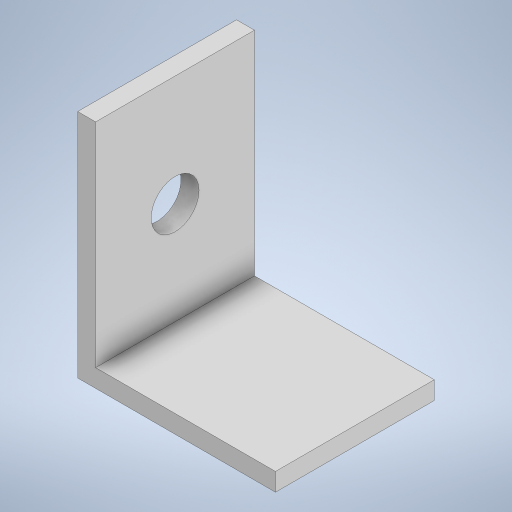
# Autodesk Inventor part: MotorHalterNeu
Saved by Autodesk Inventor 2023 (Build 270158000, 158)
## iProperties
Created: 2024-02-23
Part Number: MotorHalterNeu
Material: Generisch
Document SubType Name: Modeling
Designer: phili
Density: 1 g/cm^3
Appearance: Vorgabe
Author: phili
Autodesk Inventor part; units mm, degrees
ref_plane "YZ Plane" through (0, 0, 0) normal (1, 0, 0) x (0, 1, 0)
ref_plane "XZ Plane" through (0, 0, 0) normal (0, 1, 0) x (-1, 0, 0)
ref_plane "XY Plane" through (0, 0, 0) normal (0, 0, 1) x (1, 0, 0)
sketch "Skizze1" plane through (0, 0, 0) normal (1, 0, 0) x (0, 1, 0)
  line L0 (-19.25, -13.25) -> (19.25, -13.25)
  line L1 (19.25, -13.25) -> (19.25, 13.25)
  line L2 (19.25, 13.25) -> (-19.25, 13.25)
  line L3 (-19.25, 13.25) -> (-19.25, -13.25)
  line L4 (-19.25, -13.25) -> (19.25, 13.25) construction
  line L5 (19.25, -13.25) -> (-19.25, 13.25) construction
  point P0 (0, 0)
  dimension "d0" = 38.5
  dimension "d1" = 26.5
  constraints: 12 end point, 2 midpoint, 2 parallel, 1 horizontal, 1 perpendicular
  measures "d0" distance of L2.end L1.end
  measures "d1" distance of L1.end L0.end
extrude "Extrusion1" add sketch "Skizze1" along normal blind 33
sketch "Skizze2" plane through (0, -19.25, 13.25) normal (0, 0, 1) x (1, 0, 0)
  line L0 (0, 38.5) -> (33, 38.5) projected
  line L1 (3, 38.5) -> (33, 38.5)
  line L2 (33, 38.5) -> (33, 3)
  line L3 (33, 3) -> (3, 3)
  line L4 (3, 3) -> (3, 38.5)
  point P0 (0, 19.25)
  dimension "d4" = 35.5
  constraints: 8 end point, 2 parallel, 1 horizontal, 1 perpendicular, 1 point on line
  measures "d4" distance of L1.end L2.end
extrude "Extrusion2" cut sketch "Skizze2" against normal through all
sketch "Skizze3" plane through (0, 0, 0) normal (-1, 0, 0) x (0, 0, 1)
  line L0 (13.25, -16.25) -> (-13.25, -16.25) projected
  point P0 (0, 0)
  point P1 (0, 0.75)
  dimension "d14" = 0
  dimension "d15" = 17
  measures "d14" horizontal distance of point (0, 0) point (0, 0.75)
  measures "d15" distance from line of L0 point (0, 0.75)
hole "Bohrung1" at (0, 0.75, 0) direction (1, 0, 0) diameter 8 end through all
